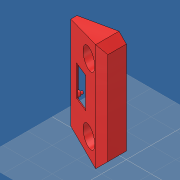
# Autodesk Inventor part: DayLightGlow_DisplayPanel_096
Saved by Autodesk Inventor 2019 (Build 230136000, 136)
## iProperties
Created: 2019-01-06
Part Number: DayLightGlow_DisplayPanel_096
Material: Generisch
Document SubType Name: Modeling
Designer: Stefan
Mass: 11.8297 g
Surface Area: 138.821 cm^2
Volume: 11.8297 cm^3
Density: 1 g/cm^3
Appearance: Hellrot
Author: Stefan
Autodesk Inventor part; units mm, degrees
ref_plane "YZ Plane" through (0, 0, 0) normal (1, 0, 0) x (0, 1, 0)
ref_plane "XZ Plane" through (0, 0, 0) normal (0, 1, 0) x (-1, 0, 0)
ref_plane "XY Plane" through (0, 0, 0) normal (0, 0, 1) x (1, 0, 0)
sketch "Skizze2" plane through (0, 0, 0) normal (0, 1, 0) x (-1, 0, 0)
  line L0 (40, 5) -> (6, 18.8682)
  line L1 (0, 0) -> (40, 0)
  line L2 (40, 5) -> (40, 0)
  line L3 (6, 18.8682) -> (0, 15)
  line L4 (0, 15) -> (0, 0)
  line L5 (0, 15) -> (0, 21.3156)
  line L6 (0, 21.3156) -> (6, 18.8682)
  line L7 (6, 18.8682) -> (0, 15)
  dimension "d0" = 40
  dimension "d40" = 5
  dimension "d43" = 15
  dimension "d45" = 6
  dimension "d46" = 125
  constraints: 16 end point, 3 vertical, 1 collinear, 1 perpendicular
  measures "d0" distance of L1.end L1.start
  measures "d40" distance of L0.start L1.end
  measures "d43" distance of L3.end L1.start
  measures "d45" distance from line of L4 L0.end
  measures "d46" angle of L3 L0
extrude "Extrusion1" add sketch "Skizze2" along normal mid plane 75 contours L2 L1 L4 L3 L0
shell "Wandung1" thickness 1.2 removed faces 1 at (-26.6667, 12.5, 0)
sketch "Skizze3" plane through (-2.2903, -36.3, 19.0854) normal (0.3776791, 0, -0.9259365) x (-0.9259365, 0, -0.3776791)
  line L0 (13.3416, 49.675) -> (13.3416, 22.925)
  line L1 (13.3416, 22.925) -> (32.6416, 22.925)
  line L2 (32.6416, 22.925) -> (32.6416, 49.675)
  line L3 (32.6416, 49.675) -> (13.3416, 49.675)
  line L4 (37.1416, 50.175) -> (37.1416, 22.425)
  line L5 (37.1416, 22.425) -> (9.1416, 22.425)
  line L6 (9.1416, 22.425) -> (9.1416, 50.175)
  line L7 (9.1416, 50.175) -> (37.1416, 50.175)
  circle A0 centre (34.8916, 48.05) radius 1
  circle A1 centre (34.8916, 24.55) radius 1
  circle A2 centre (11.3916, 48.05) radius 1
  circle A3 centre (11.3916, 24.55) radius 1
  line L8 (39.43, 0) -> (39.43, 72.6) projected
  line L9 (4.1416, 0) -> (4.1416, 72.6) projected
  line L10 (9.1416, 36.3) -> (37.1416, 36.3) construction
  circle A4 centre (34.8916, 48.05) radius 2
  circle A5 centre (34.8916, 24.55) radius 2
  circle A6 centre (11.3916, 24.55) radius 2
  circle A7 centre (11.3916, 48.05) radius 2
  line L11 (31.6416, 48.675) -> (18.3416, 48.675)
  line L12 (18.3416, 48.675) -> (18.3416, 23.925)
  line L13 (18.3416, 23.925) -> (31.6416, 23.925)
  line L14 (31.6416, 23.925) -> (31.6416, 48.675)
  point P0 (39.43, 36.3)
  dimension "d12" = 27.75
  dimension "d13" = 2
  dimension "d66" = 28
  dimension "d67" = 19.3
  dimension "d68" = 26.75
  dimension "d69" = 23.5
  dimension "d70" = 23.5
  dimension "d71" = 2.25
  dimension "d72" = 2.25
  dimension "d73" = 4.5
  dimension "d74" = 4
  dimension "d93" = 5
  dimension "d94" = 1
  dimension "d95" = 1
  dimension "d96" = 5
  constraints: 26 end point, 8 centre point, 6 equal radius, 6 parallel, 4 coincident, 3 midpoint, 3 perpendicular, 2 horizontal alignment, 2 vertical alignment, 1 horizontal, 1 point on line, 1 symmetric about line, 2 other
  measures "d12" distance of L4.start L4.end
  measures "d13" diameter of A0
  measures "d66" distance between parallel lines of L6 L4
  measures "d67" distance of L2.end L0.start
  measures "d68" distance of L1.end L2.end
  measures "d69" distance of A1.centre A0.centre
  measures "d70" distance of A0.centre A2.centre
  measures "d71" distance from line of L4 A0.centre
  measures "d72" distance from line of A2.centre L6
  measures "d73" distance between parallel lines of L4 L2
  measures "d74" diameter of A4
  measures "d93" distance between parallel lines of L0 L12
  measures "d94" distance between parallel lines of L11 L3
  measures "d95" distance between parallel lines of L14 L2
  measures "d96" distance between parallel lines of L9 L6
extrude "Extrusion2" cut sketch "Skizze3" against normal through all contours L14 L13 L12 L11
extrude "Extrusion4" add sketch "Skizze3" along normal blind 2 contours A7 L0 | L0 A7 | A6 L0 | L0 A6 | A4 | A5
extrude "Extrusion11" add sketch "Skizze3" along normal blind 4 contours A0 | A1 | A2 | A3
extrude "Extrusion15" cut sketch "Skizze3" against normal blind 0.5 contours L3 L2 L1 L0 A6 A7 | A7 L0 | A6 L0 | L14 L13 L12 L11 picked at (13.3508, 48.1492) picked at (13.3508, 24.6492)
sketch "Skizze5" plane through (0, 37.5, 0) normal (0, 0, -1) x (-1, 0, 0)
  line L0 (40, -75) -> (40, 0) projected
  line L1 (0, 0) -> (0, -75) projected
  circle A0 centre (15.2, -10.2) radius 8
  circle A1 centre (15.2, -64.8) radius 8
  circle A2 centre (15.2, -10.2) radius 9
  circle A3 centre (15.2, -64.8) radius 9
  line L2 (40, -37.5) -> (0, -37.5) construction
  line L3 (38.8, -1.2) -> (31.8, -1.2)
  line L4 (31.8, -1.2) -> (31.8, -6.2)
  line L5 (31.8, -6.2) -> (38.8, -6.2)
  line L6 (38.8, -6.2) -> (38.8, -1.2)
  line L7 (38.8, -73.8) -> (31.8, -73.8)
  line L8 (31.8, -73.8) -> (31.8, -68.8)
  line L9 (31.8, -68.8) -> (38.8, -68.8)
  line L10 (38.8, -68.8) -> (38.8, -73.8)
  line L11 (1.2, -73.8) -> (1.2, -1.2) projected
  line L12 (1.2, -1.2) -> (6.2, -1.2)
  line L13 (6.2, -1.2) -> (6.2, -6.2)
  line L14 (6.2, -6.2) -> (1.2, -6.2)
  line L15 (1.2, -6.2) -> (1.2, -1.2)
  line L16 (1.2, -73.8) -> (6.2, -73.8)
  line L17 (6.2, -73.8) -> (6.2, -68.8)
  line L18 (6.2, -68.8) -> (1.2, -68.8)
  line L19 (1.2, -68.8) -> (1.2, -73.8)
  line L20 (1.2, -1.2) -> (6.2, -6.2) construction
  line L21 (1.2, -73.8) -> (6.2, -68.8) construction
  line L22 (1.2, -1.2) -> (38.8, -1.2) projected
  line L23 (34.3, -6.2) -> (34.3, -1.2) construction
  line L24 (34.3, -68.8) -> (34.3, -73.8) construction
  point P0 (34.3, -71.3)
  point P1 (34.3, -3.7)
  point P2 (3.7, -3.7)
  point P3 (3.7, -71.3)
  point P4 (34.3, -71.3)
  point P5 (34.3, -3.7)
  dimension "d30" = 16
  dimension "d38" = 1
  dimension "d47" = 7
  dimension "d48" = 5
  dimension "d56" = 5
  dimension "d63" = 2.5
  dimension "d77" = 14
  constraints: 42 end point, 8 parallel, 7 perpendicular, 6 collinear, 5 midpoint, 4 centre point, 4 coincident, 4 horizontal, 2 equal radius, 1 symmetric about line, 1 tangent
  measures "d30" diameter of A0
  measures "d38" radial gap between concentric circles of A0 A2
  measures "d47" distance of L4.end L5.end
  measures "d48" distance of L3.end L4.end
  measures "d56" distance between parallel lines of L11 L13
  measures "d63" distance between parallel lines of L4 L23
  measures "d77" distance from line of A2.centre L11
extrude "Extrusion7" cut sketch "Skizze5" against normal up to surface contours A0 | A1 surface through (-40, 0, 5) normal (-0.3776791, 0, 0.9259365)
extrude "Extrusion8" add sketch "Skizze5" against normal up to surface contours A2 | A3 | L6 L5 L4 L3 | L7 L8 L9 L10 surface through (-39.5468, 0, 3.8889) normal (-0.3776791, 0, 0.9259365)
extrude "Extrusion10" add sketch "Skizze5" against normal up to surface contours L11 L18 L17 L16 | L11 L12 L13 L14 surface through (-6.6502, 0, 17.8597) normal (0.541855, 0, 0.840472)
hole "Bohrung1" at (-34.3, -33.8, 0) at (-34.3, 33.8, 0) at (-3.7, 33.8, 0) at (-3.7, -33.8, 0) direction (0, 0, 1) diameter 2.2 depth 6
sketch "Skizze6" plane through (0, 0, 0) normal (0, 0, 1) x (1, 0, 0)
  circle A0 centre (-3.7, 33.8) radius 1.1 projected
  circle A1 centre (-34.3, -33.8) radius 1.1 projected
  circle A2 centre (-34.3, 33.8) radius 1.1 projected
  circle A3 centre (-3.7, -33.8) radius 1.1 projected
  line L0 (-31.8, -36.3) -> (-15.2, -36.3) projected
  line L1 (-15.2, -36.3) -> (-6.2, -36.3) projected
  line L2 (-6.2, -36.3) -> (-6.2, -31.3) projected
  line L3 (-6.2, -31.3) -> (-1.2, -31.3) projected
  line L4 (-1.2, -31.3) -> (-1.2, 31.3) projected
  line L5 (-1.2, 31.3) -> (-6.2, 31.3) projected
  line L6 (-6.2, 31.3) -> (-6.2, 36.3) projected
  line L7 (-6.2, 36.3) -> (-15.2, 36.3) projected
  line L8 (-15.2, 36.3) -> (-31.8, 36.3) projected
  line L9 (-31.8, 36.3) -> (-31.8, 31.3) projected
  line L10 (-31.8, 31.3) -> (-38.8, 31.3) projected
  line L11 (-38.8, 31.3) -> (-38.8, -31.3) projected
  line L12 (-38.8, -31.3) -> (-31.8, -31.3) projected
  line L13 (-31.8, -31.3) -> (-31.8, -36.3) projected
  line L14 (-40, -37.5) -> (-40, 37.5) projected
  line L15 (0, 37.5) -> (-40, 37.5) projected
  line L16 (0, 37.5) -> (0, -37.5) projected
  line L17 (-40, -37.5) -> (0, -37.5) projected
  line L18 (-40, 37.5) -> (-6, 43.4988)
  line L19 (-6, 43.4988) -> (0, 37.5)
  line L20 (0, 37.5) -> (0, 37.5)
  line L21 (-40, 37.5) -> (0, 37.5)
  line L22 (-48, 0) -> (8, 0) projected
  line L23 (0, -37.5) -> (-40, -37.5)
  line L24 (-40, -37.5) -> (-6, -43.4988)
  line L25 (-6, -43.4988) -> (0, -37.5)
  line L26 (0, -37.5) -> (0, -37.5)
  point P0 (0, 0)
  dimension "d80" = 6
  dimension "d81" = 125
  dimension "d82" = 0
  constraints: 16 end point, 2 symmetric about line, 1 horizontal, 1 vertical
  measures "d80" distance from line of L20 L18.end
  measures "d81" angle of L19 L18
  measures "d82" distance of L19.end L15.start
extrude "Extrusion12" add sketch "Skizze6" along normal up to surface contours L17 L25 L24 | L18 L19 L15 surface through (-40, 0, 5) normal (-0.3776791, 0, 0.9259365)
extrude "Extrusion14" cut sketch "Skizze2" along normal through all both and the other way through all contours L3 L5 L6
fillet "Rundung1" [suppressed]
